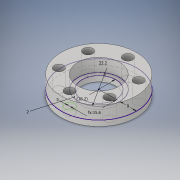
# Autodesk Inventor part: Csapagyhaz
Saved by Autodesk Inventor 2019 (Build 230136000, 136)
## iProperties
Created: 2020-02-01
Part Number: Csapagyhaz
Material: Generic
Document SubType Name: Modeling
Designer: laca
Density: 1 g/cm^3
Appearance: Default
Author: laca
Autodesk Inventor part; units mm, degrees
ref_plane "YZ Plane" through (0, 0, 0) normal (1, 0, 0) x (0, 1, 0)
ref_plane "XZ Plane" through (0, 0, 0) normal (0, 1, 0) x (-1, 0, 0)
ref_plane "XY Plane" through (0, 0, 0) normal (0, 0, 1) x (1, 0, 0)
sketch "Sketch1" plane through (0, 0, 0) normal (0, 1, 0) x (-1, 0, 0)
  circle A0 centre (0, 0) radius 11.1
  circle A1 centre (0, 0) radius 20.1
  circle A2 centre (0, 15.6) radius 2.5
  circle A3 centre (0, 0) radius 9.1
  dimension "d0" = 22.2
  dimension "d1" = 9
  dimension "d3" = 5
  dimension "d4" = 15.6
  dimension "d9" = 2
  dimension "d17" = 18.2
  constraints: 4 centre point, 2 coincident
  measures "d0" diameter of A0
  measures "d1" radial gap between concentric circles of A0 A1
  measures "d3" diameter of A2
  measures "d4" distance of A0.centre A2.centre
  measures "d9" radial gap between concentric circles of A0 A3
  measures "d17" diameter of A3
extrude "Extrusion1" add sketch "Sketch1" along normal blind 7 contours A1 | A2
extrude "Extrusion3" add sketch "Sketch1" against normal blind 3 contours A0 | A1 | A2
extrude "Extrusion4" cut sketch "Sketch1" along normal through all both and the other way through all contours A2
pattern_circular "Circular Pattern1" count 6 over 360 about axis through (0, 0, 0) along (0, -1, 0) of "Extrusion4"
equation "\"d4\" = 0.5 * d1 + 0.5 * d0"
body "Solid1"
